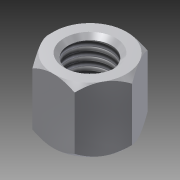
# Autodesk Inventor part: T10x2 nakretka
Saved by Autodesk Inventor 2013 (Build 170138000, 138)
## iProperties
Created: 2014-01-22
Part Number: T10x2 nakretka
Material: Generic
Document SubType Name: Modeling
Designer: Masta
Density: 1 g/cm^3
Author: Masta
Autodesk Inventor part; units mm, degrees
ref_plane "YZ Plane" through (0, 0, 0) normal (1, 0, 0) x (0, 1, 0)
ref_plane "XZ Plane" through (0, 0, 0) normal (0, 1, 0) x (-1, 0, 0)
ref_plane "XY Plane" through (0, 0, 0) normal (0, 0, 1) x (1, 0, 0)
sketch "Sketch1" plane through (0, 0, 0) normal (0, 0, 1) x (1, 0, 0)
  circle A0 centre (0, 0) radius 5
  line L0 (4.9075, 8.5) -> (9.815, 0)
  line L1 (9.815, 0) -> (4.9075, -8.5)
  line L2 (4.9075, -8.5) -> (-4.9075, -8.5)
  line L3 (-4.9075, -8.5) -> (-9.815, 0)
  line L4 (-9.815, 0) -> (-4.9075, 8.5)
  line L5 (-4.9075, 8.5) -> (4.9075, 8.5)
  dimension "d0" = 10
  dimension "d1" = 17
  constraints: 12 end point, 2 coincident, 1 centre point, 13 other
  measures "d0" diameter of A0
  measures "d1" distance between parallel lines of L5 L2
extrude "Extrusion1" add sketch "Sketch1" along normal blind 15
sketch "Sketch2" plane through (0, 0, 0) normal (1, 0, 0) x (0, 1, 0)
  line L0 (-8.5, 0) -> (-8.5, 15) projected
  line L1 (-8.5, 15) -> (-5, 15) projected
  line L2 (-5, 15) -> (-5, 0) projected
  line L3 (-5, 0) -> (-8.5, 0) projected
  line L4 (8.5, 15) -> (8.5, 0) projected
  line L5 (8.5, 0) -> (5, 0) projected
  line L6 (5, 0) -> (5, 15) projected
  line L7 (5, 15) -> (8.5, 15) projected
  line L8 (5, 14) -> (6, 15)
  line L9 (5, 14) -> (6.4142, 14) construction
  line L10 (8.5, 15) -> (12.5, 11)
  line L11 (8.5, 15) -> (14.1569, 15) construction
  line L12 (6, 15) -> (8.5, 15)
  line L13 (0, -3) -> (0, 18) projected
  line L14 (5, 7.5) -> (8.5, 7.5) construction
  line L15 (5, 0) -> (8.5, 0)
  line L16 (5, 1) -> (6, 0)
  line L17 (5, 1) -> (6.4142, 1) construction
  line L18 (8.5, 0) -> (12.5, 4)
  line L19 (8.5, 0) -> (14.1569, 0) construction
  line L20 (6, 0) -> (8.5, 0)
  line L21 (5, 14) -> (5, 1)
  line L22 (12.5, 4) -> (12.5, 11)
  point P0 (0, 0)
  dimension "d4" = 45
  dimension "d5" = 1
  dimension "d7" = 45
  dimension "d8" = 4
  constraints: 28 end point, 5 symmetric about line, 3 point on line, 2 collinear, 2 equal length, 2 horizontal, 1 midpoint, 1 parallel
  measures "d4" angle of L9 L8
  measures "d5" horizontal distance of L8.start L8.end
  measures "d7" angle of L10 L11
  measures "d8" horizontal distance of L4.start L10.end
revolve "Revolution1" cut sketch "Sketch2" angle 360 about axis through (0, 0, -10) along (0, 0, 1) keep common part contours L10 L22 L18 L4 | L4 L5 L16 L6 L8 L7
thread "Thread1" size "TR10x2" class "7H" standard "ISO Metric Trapezoidal Threads" full length
body "Solid1"
